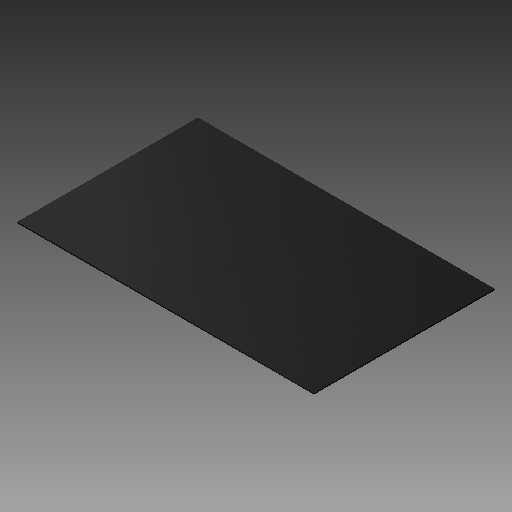
# Autodesk Inventor part: Schubladenboden
Saved by Autodesk Inventor 2018 (Build 220112000, 112)
## iProperties
Created: 2012-11-27
Part Number: Schubladenboden
Material: PVC-U
Document SubType Name: Modeling
Designer: Neef
Mass: 2378.38 g
Surface Area: 9330.5 cm^2
Volume: 1843.7 cm^3
Density: 1.29 g/cm^3
Appearance: Fine Textured - Black
Author: Neef
Autodesk Inventor part; units mm, degrees
ref_plane "YZ Plane" through (0, 0, 0) normal (1, 0, 0) x (0, 1, 0)
ref_plane "XZ Plane" through (0, 0, 0) normal (0, 1, 0) x (-1, 0, 0)
ref_plane "XY Plane" through (0, 0, 0) normal (0, 0, 1) x (1, 0, 0)
sketch "Skizze1" plane through (0, 0, 0) normal (0, 0, 1) x (1, 0, 0)
  line L0 (0, 370.86) -> (0, -370.86) projected
  line L1 (-609, 0) -> (609, 0) projected
  line L2 (435, -264.9) -> (-435, -264.9)
  line L3 (-435, -264.9) -> (-435, 264.9)
  line L4 (-435, 264.9) -> (435, 264.9)
  line L5 (435, 264.9) -> (435, -264.9)
  point P0 (0, 0)
  point P1 (0, -264.9)
  point P2 (435, 0)
  dimension "d0" = 870
  dimension "d1" = 529.8
  constraints: 8 end point, 2 midpoint, 2 parallel, 2 point on line, 1 horizontal, 1 perpendicular
  measures "d0" distance of L2.start L2.end
  measures "d1" distance of L2.end L3.end
extrude "Extrusion1" add sketch "Skizze1" along normal blind 4
